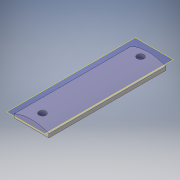
# Autodesk Inventor part: Beacon Push Bar
Saved by Autodesk Inventor 2016 (Build 200138000, 138)
## iProperties
Created: 2016-12-14
Part Number: Beacon Push Bar
Material: Generic
Document SubType Name: Modeling
Designer: paul_
Density: 1 g/cm^3
Appearance: Default
Author: paul_
Autodesk Inventor part; units mm, degrees
ref_plane "YZ Plane" through (0, 0, 0) normal (1, 0, 0) x (0, 1, 0)
ref_plane "XZ Plane" through (0, 0, 0) normal (0, 1, 0) x (-1, 0, 0)
ref_plane "XY Plane" through (0, 0, 0) normal (0, 0, 1) x (1, 0, 0)
sketch "Sketch1" plane through (0, 0, 0) normal (0, 0, 1) x (1, 0, 0)
  line L0 (0, 0) -> (38.1, 0)
  arc A0 (33.6372, 3.2217) -> (3.5441, 3.2217) centre (18.5906, -30.8441) ccw
  line L1 (-11.7643, 6.3967) -> (19.5622, 6.3967) construction
  line L2 (-11.7643, 6.3967) -> (-11.7643, 0.0467) construction
  line L3 (3.5441, 3.2217) -> (3.5441, 0)
  line L4 (33.6372, 3.2217) -> (33.6372, 0)
  line L5 (3.5441, 0) -> (33.6372, 0)
  dimension "d0" = 38.1
  dimension "d1" = 6.35
  constraints: 12 end point, 2 horizontal, 2 perpendicular, 2 point on circle, 2 point on line, 1 centre point, 1 collinear, 1 tangent, 1 vertical
  measures "d0" distance of L0.start L0.end
  measures "d1" distance of L1.start L2.end
extrude "Extrusion1" add sketch "Sketch1" along normal blind 101.6
ref_plane "Work Plane1" through (18.5906, 6.3967, 0) normal (0, -1, 0) x (1, 0, 0)
sketch "Sketch5" plane through (18.5906, 6.3967, 0) normal (0, -1, 0) x (1, 0, 0)
  point P0 (-18.5906, 0)
  point P1 (0, 6.9039)
  point P2 (0, 92.1664)
hole "Hole2" at (18.5906, 6.3967, 6.9039) at (18.5906, 6.3967, 92.1664) direction (0, -1, 0) diameter 4 end through all counterbore diameter 6 counterbore depth 3
body "Solid1"
